Autodesk Fusion 360 part; units mm, degrees
note: some values were not read from the file. Chosen so that the rebuilt part matches the saved one: which bodies a step acts on.
(part 2 of 3)
  line L533 (94.7167, 51.1985) -> (89.24, 51.1985)
  line L534 (89.24, 51.1985) -> (89.24, 52.8883)
  line L535 (89.24, 52.8883) -> (94.5973, 52.8883)
  spline S121 degree 3 poles (94.5973, 52.8883) (96.971, 52.8883) (98.0717, 51.6355) (98.0717, 49.5524) knots 0 0 0 0 1 1 1 1
  spline S122 degree 3 poles (88.5239, 51.0382) (88.5239, 50.5138) (88.1791, 50.1351) (87.7017, 50.1351) knots 0 0 0 0 1 1 1 1
  spline S123 degree 3 poles (87.7017, 50.1351) (87.2243, 50.1351) (86.8796, 50.5138) (86.8796, 51.0382) knots 0 0 0 0 1 1 1 1
  spline S124 degree 3 poles (86.8796, 51.0382) (86.8796, 51.5627) (87.2243, 51.9414) (87.7017, 51.9414) knots 0 0 0 0 1 1 1 1
  spline S125 degree 3 poles (87.7017, 51.9414) (88.1791, 51.9414) (88.5239, 51.5627) (88.5239, 51.0382) knots 0 0 0 0 1 1 1 1
  spline S126 degree 3 poles (88.5239, 48.0956) (88.5239, 47.5712) (88.1791, 47.1925) (87.7017, 47.1925) knots 0 0 0 0 1 1 1 1
  spline S127 degree 3 poles (87.7017, 47.1925) (87.2243, 47.1925) (86.8796, 47.5712) (86.8796, 48.0956) knots 0 0 0 0 1 1 1 1
  spline S128 degree 3 poles (86.8796, 48.0956) (86.8796, 48.6201) (87.2243, 48.9988) (87.7017, 48.9988) knots 0 0 0 0 1 1 1 1
  spline S129 degree 3 poles (87.7017, 48.9988) (88.1791, 48.9988) (88.5239, 48.6201) (88.5239, 48.0956) knots 0 0 0 0 1 1 1 1
  line L536 (97.9126, 35.3898) -> (97.9126, 33.7728)
  line L537 (97.9126, 33.7728) -> (94.12, 33.7728)
  spline S130 degree 3 poles (94.12, 33.7728) (93.1519, 33.7728) (92.1176, 33.9331) (91.1893, 34.0059) knots 0 0 0 0 1 1 1 1
  line L538 (91.1893, 34.0059) -> (91.1893, 33.9622)
  line L539 (91.1893, 33.9622) -> (93.0326, 33.1027)
  line L540 (93.0326, 33.1027) -> (97.9126, 30.5826)
  line L541 (97.9126, 30.5826) -> (97.9126, 28.8054)
  line L542 (97.9126, 28.8054) -> (89.24, 28.8054)
  line L543 (89.24, 28.8054) -> (89.24, 30.4224)
  line L544 (89.24, 30.4224) -> (93.0061, 30.4224)
  spline S131 degree 3 poles (93.0061, 30.4224) (93.9741, 30.4224) (95.0748, 30.2621) (95.9632, 30.1893) knots 0 0 0 0 1 1 1 1
  line L545 (95.9632, 30.1893) -> (95.9632, 30.233)
  line L546 (95.9632, 30.233) -> (94.1067, 31.0925)
  line L547 (94.1067, 31.0925) -> (89.24, 33.6126)
  line L548 (89.24, 33.6126) -> (89.24, 35.3898)
  line L549 (89.24, 35.3898) -> (97.9126, 35.3898)
  line L550 (97.9126, 17.2649) -> (97.9126, 15.5751)
  line L551 (97.9126, 15.5751) -> (94.2924, 15.5751)
  line L552 (94.2924, 15.5751) -> (94.2924, 11.8313)
  line L553 (94.2924, 11.8313) -> (92.9928, 11.8313)
  line L554 (92.9928, 11.8313) -> (92.9928, 15.5751)
  line L555 (92.9928, 15.5751) -> (90.5396, 15.5751)
  line L556 (90.5396, 15.5751) -> (90.5396, 11.1758)
  line L557 (90.5396, 11.1758) -> (89.24, 11.1758)
  line L558 (89.24, 11.1758) -> (89.24, 17.2649)
  line L559 (89.24, 17.2649) -> (97.9126, 17.2649)
  line L560 (116.9551, 192.1915) -> (116.9551, 185.9421)
  line L561 (116.9551, 185.9421) -> (115.6555, 185.9421)
  line L562 (115.6555, 185.9421) -> (115.6555, 190.5017)
  line L563 (115.6555, 190.5017) -> (113.0962, 190.5017)
  line L564 (113.0962, 190.5017) -> (113.0962, 186.7579)
  line L565 (113.0962, 186.7579) -> (111.7966, 186.7579)
  line L566 (111.7966, 186.7579) -> (111.7966, 190.5017)
  line L567 (111.7966, 190.5017) -> (109.5821, 190.5017)
  line L568 (109.5821, 190.5017) -> (109.5821, 186.0878)
  line L569 (109.5821, 186.0878) -> (108.2825, 186.0878)
  line L570 (108.2825, 186.0878) -> (108.2825, 192.1915)
  line L571 (108.2825, 192.1915) -> (116.9551, 192.1915)
  line L572 (116.9551, 174.9989) -> (116.9551, 168.7058)
  line L573 (116.9551, 168.7058) -> (115.6555, 168.7058)
  line L574 (115.6555, 168.7058) -> (115.6555, 171.0075)
  line L575 (115.6555, 171.0075) -> (109.5821, 171.0075)
  line L576 (109.5821, 171.0075) -> (109.5821, 168.7058)
  line L577 (109.5821, 168.7058) -> (108.2825, 168.7058)
  line L578 (108.2825, 168.7058) -> (108.2825, 174.9989)
  line L579 (108.2825, 174.9989) -> (109.5821, 174.9989)
  line L580 (109.5821, 174.9989) -> (109.5821, 172.6973)
  line L581 (109.5821, 172.6973) -> (115.6555, 172.6973)
  line L582 (115.6555, 172.6973) -> (115.6555, 174.9989)
  line L583 (115.6555, 174.9989) -> (116.9551, 174.9989)
  line L584 (116.9551, 157.6752) -> (116.9551, 156.0583)
  line L585 (116.9551, 156.0583) -> (113.1625, 156.0583)
  spline S132 degree 3 poles (113.1625, 156.0583) (112.1944, 156.0583) (111.1601, 156.2185) (110.2318, 156.2913) knots 0 0 0 0 1 1 1 1
  line L586 (110.2318, 156.2913) -> (110.2318, 156.2476)
  line L587 (110.2318, 156.2476) -> (112.0751, 155.3882)
  line L588 (112.0751, 155.3882) -> (116.9551, 152.868)
  line L589 (116.9551, 152.868) -> (116.9551, 151.0908)
  line L590 (116.9551, 151.0908) -> (108.2825, 151.0908)
  line L591 (108.2825, 151.0908) -> (108.2825, 152.7078)
  line L592 (108.2825, 152.7078) -> (112.0486, 152.7078)
  spline S133 degree 3 poles (112.0486, 152.7078) (113.0166, 152.7078) (114.1172, 152.5475) (115.0057, 152.4747) knots 0 0 0 0 1 1 1 1
  line L593 (115.0057, 152.4747) -> (115.0057, 152.5184)
  line L594 (115.0057, 152.5184) -> (113.1492, 153.3779)
  line L595 (113.1492, 153.3779) -> (108.2825, 155.898)
  line L596 (108.2825, 155.898) -> (108.2825, 157.6752)
  line L597 (108.2825, 157.6752) -> (116.9551, 157.6752)
  spline S134 degree 3 poles (117.1142, 136.8845) (117.1142, 134.6703) (115.9472, 133.3593) (114.5416, 133.3593) knots 0 0 0 0 1 1 1 1
  spline S135 degree 3 poles (114.5416, 133.3593) (113.2818, 133.3593) (112.632, 134.2187) (112.1944, 135.4278) knots 0 0 0 0 1 1 1 1
  line L598 (112.1944, 135.4278) -> (111.7038, 136.6806)
  spline S136 degree 3 poles (111.7038, 136.6806) (111.3988, 137.5401) (111.1468, 138.3121) (110.4838, 138.3121) knots 0 0 0 0 1 1 1 1
  spline S137 degree 3 poles (110.4838, 138.3121) (109.834, 138.3121) (109.4627, 137.7003) (109.4627, 136.7971) knots 0 0 0 0 1 1 1 1
  spline S138 degree 3 poles (109.4627, 136.7971) (109.4627, 135.8357) (109.7412, 135.1656) (110.2053, 134.5246) knots 0 0 0 0 1 1 1 1
  line L599 (110.2053, 134.5246) -> (109.224, 133.6506)
  spline S139 degree 3 poles (109.224, 133.6506) (108.5477, 134.4372) (108.1233, 135.5444) (108.1233, 136.7097) knots 0 0 0 0 1 1 1 1
  spline S140 degree 3 poles (108.1233, 136.7097) (108.1233, 138.6472) (109.1842, 140.0165) (110.5633, 140.0165) knots 0 0 0 0 1 1 1 1
  spline S141 degree 3 poles (110.5633, 140.0165) (111.8364, 140.0165) (112.5127, 138.9822) (112.8707, 137.9771) knots 0 0 0 0 1 1 1 1
  line L600 (112.8707, 137.9771) -> (113.3879, 136.6806)
  spline S142 degree 3 poles (113.3879, 136.6806) (113.7459, 135.7338) (113.9581, 135.0782) (114.7272, 135.0782) knots 0 0 0 0 1 1 1 1
  spline S143 degree 3 poles (114.7272, 135.0782) (115.3372, 135.0782) (115.7749, 135.6755) (115.7749, 136.7826) knots 0 0 0 0 1 1 1 1
  spline S144 degree 3 poles (115.7749, 136.7826) (115.7749, 137.7877) (115.377, 138.7346) (114.7935, 139.4484) knots 0 0 0 0 1 1 1 1
  line L601 (114.7935, 139.4484) -> (115.8412, 140.439)
  spline S145 degree 3 poles (115.8412, 140.439) (116.6501, 139.4921) (117.1142, 138.2247) (117.1142, 136.8845) knots 0 0 0 0 1 1 1 1
  line L602 (116.9551, 123.2901) -> (116.9551, 121.4983)
  line L603 (116.9551, 121.4983) -> (114.9129, 120.3038)
  spline S146 degree 3 poles (114.9129, 120.3038) (114.462, 120.0562) (114.0244, 119.8231) (113.494, 119.5609) knots 0 0 0 0 1 1 1 1
  line L604 (113.494, 119.5609) -> (113.494, 119.5026)
  spline S147 degree 3 poles (113.494, 119.5026) (114.0244, 119.2112) (114.462, 118.9636) (114.9129, 118.7014) knots 0 0 0 0 1 1 1 1
  line L605 (114.9129, 118.7014) -> (116.9551, 117.4632)
  line L606 (116.9551, 117.4632) -> (116.9551, 115.5986)
  line L607 (116.9551, 115.5986) -> (112.5525, 118.3955)
  line L608 (112.5525, 118.3955) -> (108.2825, 115.7734)
  line L609 (108.2825, 115.7734) -> (108.2825, 117.5652)
  line L610 (108.2825, 117.5652) -> (110.2053, 118.6431)
  spline S148 degree 3 poles (110.2053, 118.6431) (110.6031, 118.8617) (111.0142, 119.0656) (111.5314, 119.3132) knots 0 0 0 0 1 1 1 1
  line L611 (111.5314, 119.3132) -> (111.5314, 119.3715)
  spline S149 degree 3 poles (111.5314, 119.3715) (111.0142, 119.6628) (110.6031, 119.8813) (110.2053, 120.1144) knots 0 0 0 0 1 1 1 1
  line L612 (110.2053, 120.1144) -> (108.2825, 121.2361)
  line L613 (108.2825, 121.2361) -> (108.2825, 123.1153)
  line L614 (108.2825, 123.1153) -> (112.4862, 120.4932)
  line L615 (112.4862, 120.4932) -> (116.9551, 123.2901)
  spline S150 degree 3 poles (112.3403, 102.8782) (111.4253, 102.5868) (110.444, 102.2955) (109.476, 102.0333) knots 0 0 0 0 1 1 1 1
  line L616 (109.476, 102.0333) -> (109.476, 101.975)
  spline S151 degree 3 poles (109.476, 101.975) (110.444, 101.7128) (111.4253, 101.4069) (112.3403, 101.1301) knots 0 0 0 0 1 1 1 1
  line L617 (112.3403, 101.1301) -> (113.4012, 100.795)
  line L618 (113.4012, 100.795) -> (113.4012, 103.2132)
  line L619 (113.4012, 103.2132) -> (112.3403, 102.8782)
  line L620 (116.9551, 106.0538) -> (116.9551, 104.3349)
  line L621 (116.9551, 104.3349) -> (114.6079, 103.592)
  line L622 (114.6079, 103.592) -> (114.6079, 100.4163)
  line L623 (114.6079, 100.4163) -> (116.9551, 99.6879)
  line L624 (116.9551, 99.6879) -> (116.9551, 97.8961)
  line L625 (116.9551, 97.8961) -> (108.2825, 100.9844)
  line L626 (108.2825, 100.9844) -> (108.2825, 102.9656)
  line L627 (108.2825, 102.9656) -> (116.9551, 106.0538)
  spline S152 degree 3 poles (107.5664, 103.4463) (107.5664, 102.9219) (107.2216, 102.5431) (106.7442, 102.5431) knots 0 0 0 0 1 1 1 1
  spline S153 degree 3 poles (106.7442, 102.5431) (106.2668, 102.5431) (105.9221, 102.9219) (105.9221, 103.4463) knots 0 0 0 0 1 1 1 1
  spline S154 degree 3 poles (105.9221, 103.4463) (105.9221, 103.9707) (106.2668, 104.3495) (106.7442, 104.3495) knots 0 0 0 0 1 1 1 1
  spline S155 degree 3 poles (106.7442, 104.3495) (107.2216, 104.3495) (107.5664, 103.9707) (107.5664, 103.4463) knots 0 0 0 0 1 1 1 1
  spline S156 degree 3 poles (107.5664, 100.5037) (107.5664, 99.9793) (107.2216, 99.6005) (106.7442, 99.6005) knots 0 0 0 0 1 1 1 1
  spline S157 degree 3 poles (106.7442, 99.6005) (106.2668, 99.6005) (105.9221, 99.9793) (105.9221, 100.5037) knots 0 0 0 0 1 1 1 1
  spline S158 degree 3 poles (105.9221, 100.5037) (105.9221, 101.0281) (106.2668, 101.4069) (106.7442, 101.4069) knots 0 0 0 0 1 1 1 1
  spline S159 degree 3 poles (106.7442, 101.4069) (107.2216, 101.4069) (107.5664, 101.0281) (107.5664, 100.5037) knots 0 0 0 0 1 1 1 1
  line L628 (116.9551, 87.929) -> (116.9551, 86.4722)
  line L629 (116.9551, 86.4722) -> (113.4542, 86.4722)
  spline S160 degree 3 poles (113.4542, 86.4722) (112.5392, 86.4722) (110.749, 86.6179) (109.9003, 86.7199) knots 0 0 0 0 1 1 1 1
  line L630 (109.9003, 86.7199) -> (109.9003, 86.6762)
  line L631 (109.9003, 86.6762) -> (111.9159, 86.0498)
  line L632 (111.9159, 86.0498) -> (114.6609, 85.0155)
  line L633 (114.6609, 85.0155) -> (114.6609, 84.0541)
  line L634 (114.6609, 84.0541) -> (111.9159, 83.0052)
  line L635 (111.9159, 83.0052) -> (109.9003, 82.3643)
  line L636 (109.9003, 82.3643) -> (109.9003, 82.3205)
  spline S161 degree 3 poles (109.9003, 82.3205) (110.749, 82.408) (112.5392, 82.5682) (113.4542, 82.5682) knots 0 0 0 0 1 1 1 1
  line L637 (113.4542, 82.5682) -> (116.9551, 82.5682)
  line L638 (116.9551, 82.5682) -> (116.9551, 81.0823)
  line L639 (116.9551, 81.0823) -> (108.2825, 81.0823)
  line L640 (108.2825, 81.0823) -> (108.2825, 82.9469)
  line L641 (108.2825, 82.9469) -> (111.664, 84.0977)
  line L642 (111.664, 84.0977) -> (112.9636, 84.4765)
  line L643 (112.9636, 84.4765) -> (112.9636, 84.5348)
  line L644 (112.9636, 84.5348) -> (111.664, 84.9281)
  line L645 (111.664, 84.9281) -> (108.2825, 86.0643)
  line L646 (108.2825, 86.0643) -> (108.2825, 87.9289)
  line L647 (108.2825, 87.9289) -> (116.9551, 87.929)
  line L648 (116.9551, 70.5179) -> (116.9551, 63.4965)
  line L649 (116.9551, 63.4965) -> (115.6555, 63.4965)
  line L650 (115.6555, 63.4965) -> (115.6555, 68.4493)
  line L651 (115.6555, 68.4493) -> (109.2107, 63.5547)
  line L652 (109.2107, 63.5547) -> (108.2825, 63.5547)
  line L653 (108.2825, 63.5547) -> (108.2825, 70.0809)
  line L654 (108.2825, 70.0809) -> (109.5688, 70.0809)
  line L655 (109.5688, 70.0809) -> (109.5688, 65.6379)
  line L656 (109.5688, 65.6379) -> (116.0268, 70.5179)
  line L657 (116.0268, 70.5179) -> (116.9551, 70.5179)
  line L658 (116.9551, 52.4804) -> (116.9551, 50.6012)
  line L659 (116.9551, 50.6012) -> (113.8785, 49.8729)
  spline S162 degree 3 poles (113.8785, 49.8729) (113.3349, 49.7418) (112.7912, 49.6689) (112.2607, 49.5815) knots 0 0 0 0 1 1 1 1
  line L660 (112.2607, 49.5815) -> (112.2607, 49.5378)
  spline S163 degree 3 poles (112.2607, 49.5378) (112.7912, 49.4795) (113.3349, 49.363) (113.8785, 49.2319) knots 0 0 0 0 1 1 1 1
  line L661 (113.8785, 49.2319) -> (116.9551, 48.489)
  line L662 (116.9551, 48.489) -> (116.9551, 46.5807)
  line L663 (116.9551, 46.5807) -> (108.2825, 45.2988)
  line L664 (108.2825, 45.2988) -> (108.2825, 47.0031)
  line L665 (108.2825, 47.0031) -> (113.3083, 47.4693)
  spline S164 degree 3 poles (113.3083, 47.4693) (114.0244, 47.5275) (114.5681, 47.5421) (115.3903, 47.5858) knots 0 0 0 0 1 1 1 1
  line L666 (115.3903, 47.5858) -> (115.3903, 47.6441)
  spline S165 degree 3 poles (115.3903, 47.6441) (114.5681, 47.7897) (114.0244, 47.9208) (113.3083, 48.1102) knots 0 0 0 0 1 1 1 1
  line L667 (113.3083, 48.1102) -> (110.497, 48.8531)
  line L668 (110.497, 48.8531) -> (110.497, 50.1205)
  line L669 (110.497, 50.1205) -> (113.3083, 50.9071)
  spline S166 degree 3 poles (113.3083, 50.9071) (114.0377, 51.0819) (114.5814, 51.213) (115.3903, 51.3733) knots 0 0 0 0 1 1 1 1
  line L670 (115.3903, 51.3733) -> (115.3903, 51.417)
  spline S167 degree 3 poles (115.3903, 51.417) (114.5814, 51.4461) (114.0377, 51.4898) (113.3083, 51.5481) knots 0 0 0 0 1 1 1 1
  line L671 (113.3083, 51.5481) -> (108.2825, 52.0288)
  line L672 (108.2825, 52.0288) -> (108.2825, 53.8351)
  line L673 (108.2825, 53.8351) -> (116.9551, 52.4804)
  line L674 (116.9551, 34.9674) -> (116.9551, 28.718)
  line L675 (116.9551, 28.718) -> (115.6555, 28.718)
  line L676 (115.6555, 28.718) -> (115.6555, 33.2775)
  line L677 (115.6555, 33.2775) -> (113.0962, 33.2775)
  line L678 (113.0962, 33.2775) -> (113.0962, 29.5337)
  line L679 (113.0962, 29.5337) -> (111.7966, 29.5337)
  line L680 (111.7966, 29.5337) -> (111.7966, 33.2775)
  line L681 (111.7966, 33.2775) -> (109.5821, 33.2775)
  line L682 (109.5821, 33.2775) -> (109.5821, 28.8637)
  line L683 (109.5821, 28.8637) -> (108.2825, 28.8637)
  line L684 (108.2825, 28.8637) -> (108.2825, 34.9674)
  line L685 (108.2825, 34.9674) -> (116.9551, 34.9674)
  line L686 (116.9551, 17.7748) -> (116.9551, 11.4817)
  line L687 (116.9551, 11.4817) -> (115.6555, 11.4817)
  line L688 (115.6555, 11.4817) -> (115.6555, 13.7834)
  line L689 (115.6555, 13.7834) -> (109.5821, 13.7834)
  line L690 (109.5821, 13.7834) -> (109.5821, 11.4817)
  line L691 (109.5821, 11.4817) -> (108.2825, 11.4817)
  line L692 (108.2825, 11.4817) -> (108.2825, 17.7748)
  line L693 (108.2825, 17.7748) -> (109.5821, 17.7748)
  line L694 (109.5821, 17.7748) -> (109.5821, 15.4731)
  line L695 (109.5821, 15.4731) -> (115.6555, 15.4731)
  line L696 (115.6555, 15.4731) -> (115.6555, 17.7748)
  line L697 (115.6555, 17.7748) -> (116.9551, 17.7748)
  line L698 (135.9976, 192.5556) -> (135.9976, 189.9627)
  spline S168 degree 3 poles (135.9976, 189.9627) (135.9976, 187.2386) (134.4991, 185.5634) (131.6215, 185.5634) knots 0 0 0 0 1 1 1 1
  spline S169 degree 3 poles (131.6215, 185.5634) (128.7572, 185.5634) (127.325, 187.2386) (127.325, 190.0501) knots 0 0 0 0 1 1 1 1
  line L699 (127.325, 190.0501) -> (127.325, 192.5556)
  line L700 (127.325, 192.5556) -> (135.9976, 192.5556)
  line L701 (134.751, 190.8658) -> (128.5715, 190.8658)
  line L702 (128.5715, 190.8658) -> (128.5715, 190.152)
  spline S170 degree 3 poles (128.5715, 190.152) (128.5715, 188.3311) (129.4997, 187.2969) (131.6215, 187.2969) knots 0 0 0 0 1 1 1 1
  spline S171 degree 3 poles (131.6215, 187.2969) (133.7565, 187.2969) (134.751, 188.3311) (134.751, 190.152) knots 0 0 0 0 1 1 1 1
  line L703 (134.751, 190.152) -> (134.751, 190.8658)
  line L704 (135.9976, 174.9989) -> (135.9976, 173.3091)
  line L705 (135.9976, 173.3091) -> (132.6028, 173.3091)
  line L706 (132.6028, 173.3091) -> (132.6028, 171.8815)
  line L707 (132.6028, 171.8815) -> (135.9976, 169.8421)
  line L708 (135.9976, 169.8421) -> (135.9976, 167.9338)
  line L709 (135.9976, 167.9338) -> (132.3773, 170.2063)
  spline S172 degree 3 poles (132.3773, 170.2063) (132.0193, 169.07) (131.2104, 168.3125) (129.8976, 168.3125) knots 0 0 0 0 1 1 1 1
  spline S173 degree 3 poles (129.8976, 168.3125) (127.9615, 168.3125) (127.325, 169.8421) (127.325, 171.8232) knots 0 0 0 0 1 1 1 1
  line L710 (127.325, 171.8232) -> (127.325, 174.9989)
  line L711 (127.325, 174.9989) -> (135.9976, 174.9989)
  line L712 (131.3828, 173.3091) -> (128.5582, 173.3091)
  line L713 (128.5582, 173.3091) -> (128.5582, 171.998)
  spline S174 degree 3 poles (128.5582, 171.998) (128.5582, 170.687) (128.903, 169.9732) (129.8976, 169.9732) knots 0 0 0 0 1 1 1 1
  spline S175 degree 3 poles (129.8976, 169.9732) (130.8789, 169.9732) (131.3828, 170.687) (131.3828, 171.998) knots 0 0 0 0 1 1 1 1
  line L714 (131.3828, 171.998) -> (131.3828, 173.3091)
  line L715 (135.9976, 157.2528) -> (135.9976, 151.0034)
  line L716 (135.9976, 151.0034) -> (134.698, 151.0034)
  line L717 (134.698, 151.0034) -> (134.698, 155.563)
  line L718 (134.698, 155.563) -> (132.1386, 155.563)
  line L719 (132.1386, 155.563) -> (132.1386, 151.8192)
  line L720 (132.1386, 151.8192) -> (130.8391, 151.8192)
  line L721 (130.8391, 151.8192) -> (130.8391, 155.563)
  line L722 (130.8391, 155.563) -> (128.6245, 155.563)
  line L723 (128.6245, 155.563) -> (128.6245, 151.1491)
  line L724 (128.6245, 151.1491) -> (127.325, 151.1491)
  line L725 (127.325, 151.1491) -> (127.325, 157.2528)
  line L726 (127.325, 157.2528) -> (135.9976, 157.2528)
  line L727 (135.9976, 140.0602) -> (135.9976, 133.7672)
  line L728 (135.9976, 133.7672) -> (134.698, 133.7672)
  line L729 (134.698, 133.7672) -> (134.698, 136.0688)
  line L730 (134.698, 136.0688) -> (128.6245, 136.0688)
  line L731 (128.6245, 136.0688) -> (128.6245, 133.7672)
  line L732 (128.6245, 133.7672) -> (127.325, 133.7672)
  line L733 (127.325, 133.7672) -> (127.325, 140.0602)
  line L734 (127.325, 140.0602) -> (128.6245, 140.0602)
  line L735 (128.6245, 140.0602) -> (128.6245, 137.7586)
  line L736 (128.6245, 137.7586) -> (134.698, 137.7586)
  line L737 (134.698, 137.7586) -> (134.698, 140.0602)
  line L738 (134.698, 140.0602) -> (135.9976, 140.0602)
  spline S176 degree 3 poles (131.3828, 120.3475) (130.4678, 120.0562) (129.4865, 119.7648) (128.5185, 119.5026) knots 0 0 0 0 1 1 1 1
  line L739 (128.5185, 119.5026) -> (128.5185, 119.4443)
  spline S177 degree 3 poles (128.5185, 119.4443) (129.4865, 119.1821) (130.4678, 118.8762) (131.3828, 118.5994) knots 0 0 0 0 1 1 1 1
  line L740 (131.3828, 118.5994) -> (132.4437, 118.2644)
  line L741 (132.4437, 118.2644) -> (132.4437, 120.6825)
  line L742 (132.4437, 120.6825) -> (131.3828, 120.3475)
  line L743 (135.9976, 123.5232) -> (135.9976, 121.8042)
  line L744 (135.9976, 121.8042) -> (133.6504, 121.0613)
  line L745 (133.6504, 121.0613) -> (133.6504, 117.8856)
  line L746 (133.6504, 117.8856) -> (135.9976, 117.1573)
  line L747 (135.9976, 117.1573) -> (135.9976, 115.3655)
  line L748 (135.9976, 115.3655) -> (127.325, 118.4538)
  line L749 (127.325, 118.4538) -> (127.325, 120.4349)
  line L750 (127.325, 120.4349) -> (135.9976, 123.5232)
  spline S178 degree 3 poles (136.1567, 101.9604) (136.1567, 99.8627) (135.0561, 98.6537) (132.6823, 98.6537) knots 0 0 0 0 1 1 1 1
  line L751 (132.6823, 98.6537) -> (127.325, 98.6537)
  line L752 (127.325, 98.6537) -> (127.325, 100.2706)
  line L753 (127.325, 100.2706) -> (132.8017, 100.2706)
  spline S179 degree 3 poles (132.8017, 100.2706) (134.2206, 100.2706) (134.8173, 100.9261) (134.8173, 101.9604) knots 0 0 0 0 1 1 1 1
  spline S180 degree 3 poles (134.8173, 101.9604) (134.8173, 102.9801) (134.2206, 103.6065) (132.8017, 103.6065) knots 0 0 0 0 1 1 1 1
  line L754 (132.8017, 103.6065) -> (127.325, 103.6065)
  line L755 (127.325, 103.6065) -> (127.325, 105.2963)
  line L756 (127.325, 105.2963) -> (132.6823, 105.2963)
  spline S181 degree 3 poles (132.6823, 105.2963) (135.056, 105.2963) (136.1567, 104.0435) (136.1567, 101.9604) knots 0 0 0 0 1 1 1 1
  spline S182 degree 3 poles (136.1567, 84.8844) (136.1567, 82.3788) (134.7908, 81.5194) (133.1332, 81.5194) knots 0 0 0 0 1 1 1 1
  line L757 (133.1332, 81.5194) -> (127.325, 81.5194)
  line L758 (127.325, 81.5194) -> (127.325, 87.0695)
  line L759 (127.325, 87.0695) -> (128.6113, 87.0695)
  line L760 (128.6113, 87.0695) -> (128.6113, 83.2092)
  line L761 (128.6113, 83.2092) -> (133.0006, 83.2092)
  spline S183 degree 3 poles (133.0006, 83.2092) (134.3135, 83.2092) (134.8174, 83.7627) (134.8174, 84.9281) knots 0 0 0 0 1 1 1 1
  spline S184 degree 3 poles (134.8174, 84.9281) (134.8174, 85.6128) (134.4726, 86.312) (133.7698, 86.8656) knots 0 0 0 0 1 1 1 1
  line L762 (133.7698, 86.8656) -> (134.7245, 87.8561)
  spline S185 degree 3 poles (134.7245, 87.8561) (135.7456, 87.1132) (136.1567, 85.9333) (136.1567, 84.8844) knots 0 0 0 0 1 1 1 1
  line L763 (135.9976, 68.0269) -> (135.9976, 66.0312)
  line L764 (135.9976, 66.0312) -> (127.325, 63.074)
  line L765 (127.325, 63.074) -> (127.325, 64.8075)
  line L766 (127.325, 64.8075) -> (131.6878, 66.1331)
  spline S186 degree 3 poles (131.6878, 66.1331) (132.6691, 66.4245) (133.5178, 66.643) (134.5123, 66.9635) knots 0 0 0 0 1 1 1 1
  line L767 (134.5123, 66.9635) -> (134.5123, 67.0218)
  spline S187 degree 3 poles (134.5123, 67.0218) (133.5178, 67.3422) (132.6691, 67.5608) (131.6878, 67.8667) knots 0 0 0 0 1 1 1 1
  line L768 (131.6878, 67.8667) -> (127.325, 69.2068)
  line L769 (127.325, 69.2068) -> (127.325, 70.9986)
  line L770 (127.325, 70.9986) -> (135.9976, 68.0269)
  line L771 (135.9976, 52.7135) -> (135.9976, 46.4204)
  line L772 (135.9976, 46.4204) -> (134.698, 46.4204)
  line L773 (134.698, 46.4204) -> (134.698, 48.7221)
  line L774 (134.698, 48.7221) -> (128.6245, 48.7221)
  line L775 (128.6245, 48.7221) -> (128.6245, 46.4204)
  line L776 (128.6245, 46.4204) -> (127.325, 46.4204)
  line L777 (127.325, 46.4204) -> (127.325, 52.7135)
  line L778 (127.325, 52.7135) -> (128.6245, 52.7135)
  line L779 (128.6245, 52.7135) -> (128.6245, 50.4119)
  line L780 (128.6245, 50.4119) -> (134.698, 50.4119)
  line L781 (134.698, 50.4119) -> (134.698, 52.7135)
  line L782 (134.698, 52.7135) -> (135.9976, 52.7135)
  line L783 (135.9976, 34.9674) -> (135.9976, 28.718)
  line L784 (135.9976, 28.718) -> (134.698, 28.718)
  line L785 (134.698, 28.718) -> (134.698, 33.2775)
  line L786 (134.698, 33.2775) -> (132.1386, 33.2775)
  line L787 (132.1386, 33.2775) -> (132.1386, 29.5337)
  line L788 (132.1386, 29.5337) -> (130.8391, 29.5337)
  line L789 (130.8391, 29.5337) -> (130.8391, 33.2775)
  line L790 (130.8391, 33.2775) -> (128.6245, 33.2775)
  line L791 (128.6245, 33.2775) -> (128.6245, 28.8637)
  line L792 (128.6245, 28.8637) -> (127.325, 28.8637)
  line L793 (127.325, 28.8637) -> (127.325, 34.9674)
  line L794 (127.325, 34.9674) -> (135.9976, 34.9674)
  line L795 (135.9976, 17.7748) -> (135.9976, 16.085)
  line L796 (135.9976, 16.085) -> (132.6028, 16.085)
  line L797 (132.6028, 16.085) -> (132.6028, 14.6574)
  line L798 (132.6028, 14.6574) -> (135.9976, 12.618)
  line L799 (135.9976, 12.618) -> (135.9976, 10.7096)
  line L800 (135.9976, 10.7096) -> (132.3773, 12.9822)
  spline S188 degree 3 poles (132.3773, 12.9822) (132.0193, 11.8459) (131.2104, 11.0884) (129.8976, 11.0884) knots 0 0 0 0 1 1 1 1
  spline S189 degree 3 poles (129.8976, 11.0884) (127.9615, 11.0884) (127.325, 12.618) (127.325, 14.5991) knots 0 0 0 0 1 1 1 1
  line L801 (127.325, 14.5991) -> (127.325, 17.7748)
  line L802 (127.325, 17.7748) -> (135.9976, 17.7748)
  line L803 (131.3828, 16.085) -> (128.5582, 16.085)
  line L804 (128.5582, 16.085) -> (128.5582, 14.7739)
  spline S190 degree 3 poles (128.5582, 14.7739) (128.5582, 13.4629) (128.903, 12.7491) (129.8976, 12.7491) knots 0 0 0 0 1 1 1 1
  spline S191 degree 3 poles (129.8976, 12.7491) (130.8789, 12.7491) (131.3828, 13.4628) (131.3828, 14.7739) knots 0 0 0 0 1 1 1 1
  line L805 (131.3828, 14.7739) -> (131.3828, 16.085)
  spline S192 degree 3 poles (155.1992, 189.2926) (155.1992, 187.0784) (154.0322, 185.7673) (152.6266, 185.7673) knots 0 0 0 0 1 1 1 1
  spline S193 degree 3 poles (152.6266, 185.7673) (151.3668, 185.7673) (150.717, 186.6268) (150.2794, 187.8358) knots 0 0 0 0 1 1 1 1
  line L806 (150.2794, 187.8358) -> (149.7888, 189.0886)
  spline S194 degree 3 poles (149.7888, 189.0886) (149.4838, 189.9481) (149.2318, 190.7202) (148.5688, 190.7202) knots 0 0 0 0 1 1 1 1
  spline S195 degree 3 poles (148.5688, 190.7202) (147.919, 190.7202) (147.5477, 190.1083) (147.5477, 189.2052) knots 0 0 0 0 1 1 1 1
  spline S196 degree 3 poles (147.5477, 189.2052) (147.5477, 188.2437) (147.8262, 187.5736) (148.2903, 186.9327) knots 0 0 0 0 1 1 1 1
  line L807 (148.2903, 186.9327) -> (147.309, 186.0586)
  spline S197 degree 3 poles (147.309, 186.0586) (146.6327, 186.8453) (146.2083, 187.9524) (146.2083, 189.1178) knots 0 0 0 0 1 1 1 1
  spline S198 degree 3 poles (146.2083, 189.1178) (146.2083, 191.0552) (147.2692, 192.4245) (148.6483, 192.4245) knots 0 0 0 0 1 1 1 1
  spline S199 degree 3 poles (148.6483, 192.4245) (149.9214, 192.4245) (150.5977, 191.3903) (150.9557, 190.3851) knots 0 0 0 0 1 1 1 1
  line L808 (150.9557, 190.3851) -> (151.4729, 189.0886)
  spline S200 degree 3 poles (151.4729, 189.0886) (151.8309, 188.1418) (152.0431, 187.4862) (152.8122, 187.4862) knots 0 0 0 0 1 1 1 1
  spline S201 degree 3 poles (152.8122, 187.4862) (153.4222, 187.4862) (153.8598, 188.0835) (153.8598, 189.1906) knots 0 0 0 0 1 1 1 1
  spline S202 degree 3 poles (153.8598, 189.1906) (153.8598, 190.1957) (153.462, 191.1426) (152.8785, 191.8564) knots 0 0 0 0 1 1 1 1
  line L809 (152.8785, 191.8564) -> (153.9262, 192.847)
  spline S203 degree 3 poles (153.9262, 192.847) (154.735, 191.9001) (155.1992, 190.6327) (155.1992, 189.2926) knots 0 0 0 0 1 1 1 1
  line L810 (155.04, 174.7221) -> (155.04, 168.4728)
  line L811 (155.04, 168.4728) -> (153.7405, 168.4728)
  line L812 (153.7405, 168.4728) -> (153.7405, 173.0323)
  line L813 (153.7405, 173.0323) -> (151.1811, 173.0323)
  line L814 (151.1811, 173.0323) -> (151.1811, 169.2885)
  line L815 (151.1811, 169.2885) -> (149.8816, 169.2885)
  line L816 (149.8816, 169.2885) -> (149.8816, 173.0323)
  line L817 (149.8816, 173.0323) -> (147.667, 173.0323)
  line L818 (147.667, 173.0323) -> (147.667, 168.6184)
  line L819 (147.667, 168.6184) -> (146.3674, 168.6184)
  line L820 (146.3674, 168.6184) -> (146.3674, 174.7221)
  line L821 (146.3674, 174.7221) -> (155.04, 174.7221)
  spline S204 degree 3 poles (155.1992, 153.5964) (155.1992, 152.329) (154.7483, 151.3239) (153.9394, 150.5664) knots 0 0 0 0 1 1 1 1
  line L822 (153.9394, 150.5664) -> (152.9979, 151.4987)
  spline S205 degree 3 poles (152.9979, 151.4987) (153.5416, 152.0377) (153.8598, 152.6641) (153.8598, 153.4362) knots 0 0 0 0 1 1 1 1
  spline S206 degree 3 poles (153.8598, 153.4362) (153.8598, 155.0677) (152.6664, 156.1457) (150.6905, 156.1457) knots 0 0 0 0 1 1 1 1
  spline S207 degree 3 poles (150.6905, 156.1457) (148.7412, 156.1457) (147.5477, 155.0677) (147.5477, 153.4799) knots 0 0 0 0 1 1 1 1
  spline S208 degree 3 poles (147.5477, 153.4799) (147.5477, 152.7369) (147.8262, 152.1688) (148.2505, 151.6881) knots 0 0 0 0 1 1 1 1
  line L823 (148.2505, 151.6881) -> (147.2957, 150.7558)
  spline S209 degree 3 poles (147.2957, 150.7558) (146.7255, 151.353) (146.2083, 152.2999) (146.2083, 153.4799) knots 0 0 0 0 1 1 1 1
  spline S210 degree 3 poles (146.2083, 153.4799) (146.2083, 156) (147.8924, 157.8792) (150.7302, 157.8792) knots 0 0 0 0 1 1 1 1
  spline S211 degree 3 poles (150.7302, 157.8792) (153.6078, 157.8792) (155.1991, 155.9563) (155.1992, 153.5964) knots 0 0 0 0 1 1 1 1
  line L824 (155.04, 140.235) -> (155.04, 138.5452)
  line L825 (155.04, 138.5452) -> (151.1944, 138.5452)
  line L826 (151.1944, 138.5452) -> (151.1944, 135.2822)
  line L827 (151.1944, 135.2822) -> (155.04, 135.2822)
  line L828 (155.04, 135.2822) -> (155.04, 133.5924)
  line L829 (155.04, 133.5924) -> (146.3675, 133.5924)
  line L830 (146.3675, 133.5924) -> (146.3675, 135.2822)
  line L831 (146.3675, 135.2822) -> (149.8551, 135.2822)
  line L832 (149.8551, 135.2822) -> (149.8551, 138.5452)
  line L833 (149.8551, 138.5452) -> (146.3675, 138.5452)
  line L834 (146.3675, 138.5452) -> (146.3675, 140.235)
  line L835 (146.3675, 140.235) -> (155.04, 140.235)
  spline S212 degree 3 poles (155.1992, 119.4152) (155.1992, 117.201) (154.0322, 115.8899) (152.6266, 115.8899) knots 0 0 0 0 1 1 1 1
  spline S213 degree 3 poles (152.6266, 115.8899) (151.3668, 115.8899) (150.717, 116.7494) (150.2794, 117.9585) knots 0 0 0 0 1 1 1 1
  line L836 (150.2794, 117.9585) -> (149.7888, 119.2113)
  spline S214 degree 3 poles (149.7888, 119.2113) (149.4838, 120.0707) (149.2318, 120.8428) (148.5688, 120.8428) knots 0 0 0 0 1 1 1 1
  spline S215 degree 3 poles (148.5688, 120.8428) (147.919, 120.8428) (147.5477, 120.231) (147.5477, 119.3278) knots 0 0 0 0 1 1 1 1
  spline S216 degree 3 poles (147.5477, 119.3278) (147.5477, 118.3664) (147.8262, 117.6963) (148.2903, 117.0553) knots 0 0 0 0 1 1 1 1
  line L837 (148.2903, 117.0553) -> (147.309, 116.1813)
  spline S217 degree 3 poles (147.309, 116.1813) (146.6327, 116.9679) (146.2083, 118.075) (146.2083, 119.2404) knots 0 0 0 0 1 1 1 1
  spline S218 degree 3 poles (146.2083, 119.2404) (146.2083, 121.1779) (147.2692, 122.5472) (148.6483, 122.5472) knots 0 0 0 0 1 1 1 1
  spline S219 degree 3 poles (148.6483, 122.5472) (149.9214, 122.5472) (150.5977, 121.5129) (150.9557, 120.5078) knots 0 0 0 0 1 1 1 1
  line L838 (150.9557, 120.5078) -> (151.4729, 119.2113)
  spline S220 degree 3 poles (151.4729, 119.2113) (151.8309, 118.2644) (152.0431, 117.6089) (152.8122, 117.6089) knots 0 0 0 0 1 1 1 1
  spline S221 degree 3 poles (152.8122, 117.6089) (153.4222, 117.6089) (153.8598, 118.2061) (153.8598, 119.3133) knots 0 0 0 0 1 1 1 1
  spline S222 degree 3 poles (153.8598, 119.3133) (153.8598, 120.3184) (153.462, 121.2653) (152.8785, 121.9791) knots 0 0 0 0 1 1 1 1
  line L839 (152.8785, 121.9791) -> (153.9262, 122.9696)
  spline S223 degree 3 poles (153.9262, 122.9696) (154.735, 122.0228) (155.1992, 120.7554) (155.1992, 119.4152) knots 0 0 0 0 1 1 1 1
  line L840 (155.04, 105.2672) -> (155.04, 103.6502)
  line L841 (155.04, 103.6502) -> (151.2474, 103.6502)
  spline S224 degree 3 poles (151.2474, 103.6502) (150.2794, 103.6502) (149.2451, 103.8105) (148.3168, 103.8833) knots 0 0 0 0 1 1 1 1
  line L842 (148.3168, 103.8833) -> (148.3168, 103.8396)
  line L843 (148.3168, 103.8396) -> (150.1601, 102.9801)
  line L844 (150.1601, 102.9801) -> (155.04, 100.46)
  line L845 (155.04, 100.46) -> (155.04, 98.6828)
  line L846 (155.04, 98.6828) -> (146.3675, 98.6828)
  line L847 (146.3675, 98.6828) -> (146.3675, 100.2997)
  line L848 (146.3675, 100.2997) -> (150.1335, 100.2997)
  spline S225 degree 3 poles (150.1335, 100.2997) (151.1016, 100.2997) (152.2022, 100.1395) (153.0907, 100.0667) knots 0 0 0 0 1 1 1 1
  line L849 (153.0907, 100.0667) -> (153.0907, 100.1104)
  line L850 (153.0907, 100.1104) -> (151.2342, 100.9699)
  line L851 (151.2342, 100.9699) -> (146.3675, 103.49)
  line L852 (146.3675, 103.49) -> (146.3675, 105.2672)
  line L853 (146.3675, 105.2672) -> (155.04, 105.2672)
  line L854 (155.04, 87.1278) -> (155.04, 80.9804)
  line L855 (155.04, 80.9804) -> (153.7405, 80.9804)
  line L856 (153.7405, 80.9804) -> (153.7405, 85.4525)
  line L857 (153.7405, 85.4525) -> (146.3675, 85.4525)
  line L858 (146.3675, 85.4525) -> (146.3675, 87.1278)
  line L859 (146.3675, 87.1278) -> (155.04, 87.1278)
  spline S226 degree 3 poles (150.4253, 67.9395) (149.5103, 67.6481) (148.529, 67.3568) (147.561, 67.0946) knots 0 0 0 0 1 1 1 1
  line L860 (147.561, 67.0946) -> (147.561, 67.0363)
  spline S227 degree 3 poles (147.561, 67.0363) (148.529, 66.7741) (149.5103, 66.4682) (150.4253, 66.1914) knots 0 0 0 0 1 1 1 1
  line L861 (150.4253, 66.1914) -> (151.4861, 65.8564)
  line L862 (151.4861, 65.8564) -> (151.4861, 68.2745)
  line L863 (151.4861, 68.2745) -> (150.4253, 67.9395)
  line L864 (155.04, 71.1152) -> (155.04, 69.3962)
  line L865 (155.04, 69.3962) -> (152.6929, 68.6533)
  line L866 (152.6929, 68.6533) -> (152.6929, 65.4776)
  line L867 (152.6929, 65.4776) -> (155.04, 64.7492)
  line L868 (155.04, 64.7492) -> (155.04, 62.9575)
  line L869 (155.04, 62.9575) -> (146.3675, 66.0457)
  line L870 (146.3675, 66.0457) -> (146.3675, 68.0269)
  line L871 (146.3675, 68.0269) -> (155.04, 71.1152)
  spline S228 degree 3 poles (155.1992, 48.7803) (155.1992, 47.513) (154.7483, 46.5078) (153.9394, 45.7503) knots 0 0 0 0 1 1 1 1
  line L872 (153.9394, 45.7503) -> (152.9979, 46.6826)
  spline S229 degree 3 poles (152.9979, 46.6826) (153.5416, 47.2216) (153.8598, 47.848) (153.8598, 48.6201) knots 0 0 0 0 1 1 1 1
  spline S230 degree 3 poles (153.8598, 48.6201) (153.8598, 50.2516) (152.6664, 51.3296) (150.6905, 51.3296) knots 0 0 0 0 1 1 1 1
  spline S231 degree 3 poles (150.6905, 51.3296) (148.7412, 51.3296) (147.5477, 50.2516) (147.5477, 48.6637) knots 0 0 0 0 1 1 1 1
  spline S232 degree 3 poles (147.5477, 48.6637) (147.5477, 47.9208) (147.8262, 47.3527) (148.2505, 46.872) knots 0 0 0 0 1 1 1 1
  line L873 (148.2505, 46.872) -> (147.2957, 45.9397)
  spline S233 degree 3 poles (147.2957, 45.9397) (146.7255, 46.5369) (146.2083, 47.4838) (146.2083, 48.6637) knots 0 0 0 0 1 1 1 1
  spline S234 degree 3 poles (146.2083, 48.6637) (146.2083, 51.1839) (147.8924, 53.0631) (150.7302, 53.0631) knots 0 0 0 0 1 1 1 1
  spline S235 degree 3 poles (150.7302, 53.0631) (153.6078, 53.0631) (155.1991, 51.1402) (155.1992, 48.7803) knots 0 0 0 0 1 1 1 1
  line L874 (155.04, 35.419) -> (155.04, 33.7292)
  line L875 (155.04, 33.7292) -> (151.1944, 33.7292)
  line L876 (151.1944, 33.7292) -> (151.1944, 30.4661)
  line L877 (151.1944, 30.4661) -> (155.04, 30.4661)
  line L878 (155.04, 30.4661) -> (155.04, 28.7763)
  line L879 (155.04, 28.7763) -> (146.3675, 28.7763)
  line L880 (146.3675, 28.7763) -> (146.3675, 30.4661)
  line L881 (146.3675, 30.4661) -> (149.8551, 30.4661)
  line L882 (149.8551, 30.4661) -> (149.8551, 33.7292)
  line L883 (149.8551, 33.7292) -> (146.3675, 33.7292)
  line L884 (146.3675, 33.7292) -> (146.3675, 35.419)
  line L885 (146.3675, 35.419) -> (155.04, 35.419)
  line L886 (155.04, 15.4732) -> (155.04, 13.7834)
  line L887 (155.04, 13.7834) -> (147.667, 13.7834)
  line L888 (147.667, 13.7834) -> (147.667, 10.7825)
  line L889 (147.667, 10.7825) -> (146.3675, 10.7825)
  line L890 (146.3675, 10.7825) -> (146.3675, 18.4741)
  line L891 (146.3675, 18.4741) -> (147.667, 18.4741)
  line L892 (147.667, 18.4741) -> (147.667, 15.4732)
  line L893 (147.667, 15.4732) -> (155.04, 15.4732)
  spline S236 degree 3 poles (174.2417, 189.2926) (174.2417, 187.0784) (173.0747, 185.7673) (171.6691, 185.7673) knots 0 0 0 0 1 1 1 1
  spline S237 degree 3 poles (171.6691, 185.7673) (170.4093, 185.7673) (169.7595, 186.6268) (169.3219, 187.8358) knots 0 0 0 0 1 1 1 1
  line L894 (169.3219, 187.8358) -> (168.8313, 189.0886)
  spline S238 degree 3 poles (168.8313, 189.0886) (168.5263, 189.9481) (168.2743, 190.7202) (167.6113, 190.7202) knots 0 0 0 0 1 1 1 1
  spline S239 degree 3 poles (167.6113, 190.7202) (166.9615, 190.7202) (166.5902, 190.1083) (166.5902, 189.2052) knots 0 0 0 0 1 1 1 1
  spline S240 degree 3 poles (166.5902, 189.2052) (166.5902, 188.2437) (166.8687, 187.5736) (167.3328, 186.9327) knots 0 0 0 0 1 1 1 1
  line L895 (167.3328, 186.9327) -> (166.3515, 186.0586)
  spline S241 degree 3 poles (166.3515, 186.0586) (165.6752, 186.8453) (165.2509, 187.9524) (165.2509, 189.1178) knots 0 0 0 0 1 1 1 1
  spline S242 degree 3 poles (165.2509, 189.1178) (165.2509, 191.0552) (166.3117, 192.4245) (167.6909, 192.4245) knots 0 0 0 0 1 1 1 1
  spline S243 degree 3 poles (167.6909, 192.4245) (168.9639, 192.4245) (169.6402, 191.3903) (169.9982, 190.3851) knots 0 0 0 0 1 1 1 1
  line L896 (169.9982, 190.3851) -> (170.5154, 189.0886)
  spline S244 degree 3 poles (170.5154, 189.0886) (170.8735, 188.1418) (171.0856, 187.4862) (171.8548, 187.4862) knots 0 0 0 0 1 1 1 1
  spline S245 degree 3 poles (171.8548, 187.4862) (172.4648, 187.4862) (172.9024, 188.0835) (172.9024, 189.1906) knots 0 0 0 0 1 1 1 1
  spline S246 degree 3 poles (172.9024, 189.1906) (172.9024, 190.1957) (172.5045, 191.1426) (171.9211, 191.8564) knots 0 0 0 0 1 1 1 1
  line L897 (171.9211, 191.8564) -> (172.9687, 192.847)
  spline S247 degree 3 poles (172.9687, 192.847) (173.7776, 191.9001) (174.2417, 190.6327) (174.2417, 189.2926) knots 0 0 0 0 1 1 1 1
  line L898 (174.0825, 174.9989) -> (174.0825, 168.7058)
  line L899 (174.0825, 168.7058) -> (172.783, 168.7058)
  line L900 (172.783, 168.7058) -> (172.783, 171.0075)
  line L901 (172.783, 171.0075) -> (166.7095, 171.0075)
  line L902 (166.7095, 171.0075) -> (166.7095, 168.7058)
  line L903 (166.7095, 168.7058) -> (165.41, 168.7058)
  line L904 (165.41, 168.7058) -> (165.41, 174.9989)
  line L905 (165.41, 174.9989) -> (166.7095, 174.9989)
  line L906 (166.7095, 174.9989) -> (166.7095, 172.6973)
  line L907 (166.7095, 172.6973) -> (172.783, 172.6973)
  line L908 (172.783, 172.6973) -> (172.783, 174.9989)
  line L909 (172.783, 174.9989) -> (174.0825, 174.9989)
  line L910 (174.0825, 157.2528) -> (174.0825, 151.0034)
  line L911 (174.0825, 151.0034) -> (172.783, 151.0034)
  line L912 (172.783, 151.0034) -> (172.783, 155.563)
  line L913 (172.783, 155.563) -> (170.2236, 155.563)
  line L914 (170.2236, 155.563) -> (170.2236, 151.8192)
  line L915 (170.2236, 151.8192) -> (168.9241, 151.8192)
  line L916 (168.9241, 151.8192) -> (168.9241, 155.563)
  line L917 (168.9241, 155.563) -> (166.7095, 155.563)
  line L918 (166.7095, 155.563) -> (166.7095, 151.1491)
  line L919 (166.7095, 151.1491) -> (165.41, 151.1491)
  line L920 (165.41, 151.1491) -> (165.41, 157.2528)
  line L921 (165.41, 157.2528) -> (174.0825, 157.2528)
  line L922 (174.0825, 140.0311) -> (174.0825, 136.8263)
  spline S248 degree 3 poles (174.0825, 136.8263) (174.0825, 134.7286) (173.2736, 133.199) (171.5365, 133.199) knots 0 0 0 0 1 1 1 1
  spline S249 degree 3 poles (171.5365, 133.199) (170.3563, 133.199) (169.6932, 133.9711) (169.481, 135.3404) knots 0 0 0 0 1 1 1 1
  line L923 (169.481, 135.3404) -> (169.428, 135.3404)
  spline S250 degree 3 poles (169.428, 135.3404) (169.1628, 134.2187) (168.3671, 133.6943) (167.545, 133.6943) knots 0 0 0 0 1 1 1 1
  spline S251 degree 3 poles (167.545, 133.6943) (165.9537, 133.6943) (165.41, 135.1074) (165.41, 137.0739) knots 0 0 0 0 1 1 1 1
  line L924 (165.41, 137.0739) -> (165.41, 140.0311)
  line L925 (165.41, 140.0311) -> (174.0825, 140.0311)
  line L926 (168.9771, 138.3413) -> (166.6432, 138.3413)
  line L927 (166.6432, 138.3413) -> (166.6432, 137.1905)
  spline S252 degree 3 poles (166.6432, 137.1905) (166.6432, 135.9522) (166.935, 135.355) (167.7306, 135.355) knots 0 0 0 0 1 1 1 1
  spline S253 degree 3 poles (167.7306, 135.355) (168.5395, 135.355) (168.9771, 135.894) (168.9771, 137.2196) knots 0 0 0 0 1 1 1 1
  line L928 (168.9771, 137.2196) -> (168.9771, 138.3413)
  line L929 (172.8493, 138.3413) -> (170.1441, 138.3413)
  line L930 (170.1441, 138.3413) -> (170.1441, 137.0011)
  spline S254 degree 3 poles (170.1441, 137.0011) (170.1441, 135.5735) (170.5154, 134.8597) (171.4304, 134.8597) knots 0 0 0 0 1 1 1 1
  spline S255 degree 3 poles (171.4304, 134.8597) (172.4117, 134.8597) (172.8493, 135.6026) (172.8493, 137.0011) knots 0 0 0 0 1 1 1 1
  line L931 (172.8493, 137.0011) -> (172.8493, 138.3413)
  line L932 (174.0825, 122.3141) -> (174.0825, 116.0647)
  line L933 (174.0825, 116.0647) -> (172.783, 116.0647)
  line L934 (172.783, 116.0647) -> (172.783, 120.6243)
  line L935 (172.783, 120.6243) -> (170.2236, 120.6243)
  line L936 (170.2236, 120.6243) -> (170.2236, 116.8805)
  line L937 (170.2236, 116.8805) -> (168.9241, 116.8805)
  line L938 (168.9241, 116.8805) -> (168.9241, 120.6243)
  line L939 (168.9241, 120.6243) -> (166.7095, 120.6243)
  line L940 (166.7095, 120.6243) -> (166.7095, 116.2104)
  line L941 (166.7095, 116.2104) -> (165.41, 116.2104)
  line L942 (165.41, 116.2104) -> (165.41, 122.3141)
  line L943 (165.41, 122.3141) -> (174.0825, 122.3141)
  line L944 (174.0825, 105.2672) -> (174.0825, 103.6502)
  line L945 (174.0825, 103.6502) -> (170.2899, 103.6502)
  spline S256 degree 3 poles (170.2899, 103.6502) (169.3219, 103.6502) (168.2876, 103.8105) (167.3593, 103.8833) knots 0 0 0 0 1 1 1 1
  line L946 (167.3593, 103.8833) -> (167.3593, 103.8396)
  line L947 (167.3593, 103.8396) -> (169.2026, 102.9801)
  line L948 (169.2026, 102.9801) -> (174.0825, 100.46)
  line L949 (174.0825, 100.46) -> (174.0825, 98.6828)
  line L950 (174.0825, 98.6828) -> (165.41, 98.6828)
  line L951 (165.41, 98.6828) -> (165.41, 100.2997)
  line L952 (165.41, 100.2997) -> (169.176, 100.2997)
  spline S257 degree 3 poles (169.176, 100.2997) (170.1441, 100.2997) (171.2447, 100.1395) (172.1332, 100.0667) knots 0 0 0 0 1 1 1 1
  line L953 (172.1332, 100.0667) -> (172.1332, 100.1104)
  line L954 (172.1332, 100.1104) -> (170.2767, 100.9699)
  line L955 (170.2767, 100.9699) -> (165.41, 103.49)
  line L956 (165.41, 103.49) -> (165.41, 105.2672)
  line L957 (165.41, 105.2672) -> (174.0825, 105.2672)
  line L958 (174.0825, 87.9872) -> (174.0825, 80.9658)
  line L959 (174.0825, 80.9658) -> (172.783, 80.9658)
  line L960 (172.783, 80.9658) -> (172.783, 85.9187)
  line L961 (172.783, 85.9187) -> (166.3382, 81.0241)
  line L962 (166.3382, 81.0241) -> (165.41, 81.0241)
  line L963 (165.41, 81.0241) -> (165.41, 87.5502)
  line L964 (165.41, 87.5502) -> (166.6963, 87.5502)
  line L965 (166.6963, 87.5502) -> (166.6963, 83.1072)
  line L966 (166.6963, 83.1072) -> (173.1543, 87.9872)
  line L967 (173.1543, 87.9872) -> (174.0825, 87.9872)
  line L968 (174.0825, 69.9498) -> (174.0825, 68.0706)
  line L969 (174.0825, 68.0706) -> (171.006, 67.3422)
  spline S258 degree 3 poles (171.006, 67.3422) (170.4623, 67.2111) (169.9187, 67.1383) (169.3882, 67.0509) knots 0 0 0 0 1 1 1 1
  line L970 (169.3882, 67.0509) -> (169.3882, 67.0072)
  spline S259 degree 3 poles (169.3882, 67.0072) (169.9187, 66.9489) (170.4623, 66.8324) (171.006, 66.7012) knots 0 0 0 0 1 1 1 1
  line L971 (171.006, 66.7012) -> (174.0825, 65.9583)
  line L972 (174.0825, 65.9583) -> (174.0825, 64.05)
  line L973 (174.0825, 64.05) -> (165.41, 62.7681)
  line L974 (165.41, 62.7681) -> (165.41, 64.4724)
  line L975 (165.41, 64.4724) -> (170.4358, 64.9386)
  spline S260 degree 3 poles (170.4358, 64.9386) (171.1519, 64.9969) (171.6956, 65.0114) (172.5178, 65.0551) knots 0 0 0 0 1 1 1 1
  line L976 (172.5178, 65.0551) -> (172.5178, 65.1134)
  spline S261 degree 3 poles (172.5178, 65.1134) (171.6956, 65.2591) (171.1519, 65.3902) (170.4358, 65.5795) knots 0 0 0 0 1 1 1 1
  line L977 (170.4358, 65.5795) -> (167.6245, 66.3225)
  line L978 (167.6245, 66.3225) -> (167.6245, 67.5898)
  line L979 (167.6245, 67.5898) -> (170.4358, 68.3765)
  spline S262 degree 3 poles (170.4358, 68.3765) (171.1652, 68.5513) (171.7088, 68.6824) (172.5178, 68.8426) knots 0 0 0 0 1 1 1 1
  line L980 (172.5178, 68.8426) -> (172.5178, 68.8863)
  spline S263 degree 3 poles (172.5178, 68.8863) (171.7088, 68.9155) (171.1652, 68.9591) (170.4358, 69.0174) knots 0 0 0 0 1 1 1 1
  line L981 (170.4358, 69.0174) -> (165.41, 69.4982)
  line L982 (165.41, 69.4982) -> (165.41, 71.3045)
  line L983 (165.41, 71.3045) -> (174.0825, 69.9498)
  spline S264 degree 3 poles (174.2417, 49.567) (174.2417, 47.3528) (172.6106, 45.8232) (169.7065, 45.8232) knots 0 0 0 0 1 1 1 1
  spline S265 degree 3 poles (169.7065, 45.8232) (166.8554, 45.8232) (165.2508, 47.3527) (165.2508, 49.567) knots 0 0 0 0 1 1 1 1
  spline S266 degree 3 poles (165.2508, 49.567) (165.2508, 51.7812) (166.8554, 53.3108) (169.7065, 53.3108) knots 0 0 0 0 1 1 1 1
  spline S267 degree 3 poles (169.7065, 53.3108) (172.6106, 53.3108) (174.2417, 51.7812) (174.2417, 49.567) knots 0 0 0 0 1 1 1 1
  spline S268 degree 3 poles (172.9023, 49.567) (172.9023, 50.7906) (171.7486, 51.5772) (169.7065, 51.5772) knots 0 0 0 0 1 1 1 1
  spline S269 degree 3 poles (169.7065, 51.5772) (167.7174, 51.5772) (166.5902, 50.7906) (166.5902, 49.567) knots 0 0 0 0 1 1 1 1
  spline S270 degree 3 poles (166.5902, 49.567) (166.5902, 48.3433) (167.7174, 47.5567) (169.7065, 47.5567) knots 0 0 0 0 1 1 1 1
  spline S271 degree 3 poles (169.7065, 47.5567) (171.7486, 47.5567) (172.9023, 48.3433) (172.9023, 49.567) knots 0 0 0 0 1 1 1 1
  spline S272 degree 3 poles (164.6939, 51.0383) (164.6939, 50.5139) (164.3491, 50.1351) (163.8717, 50.1351) knots 0 0 0 0 1 1 1 1
  spline S273 degree 3 poles (163.8717, 50.1351) (163.3943, 50.1351) (163.0495, 50.5139) (163.0495, 51.0383) knots 0 0 0 0 1 1 1 1
  spline S274 degree 3 poles (163.0495, 51.0383) (163.0495, 51.5627) (163.3943, 51.9414) (163.8717, 51.9414) knots 0 0 0 0 1 1 1 1
  spline S275 degree 3 poles (163.8717, 51.9414) (164.3491, 51.9414) (164.6939, 51.5627) (164.6939, 51.0383) knots 0 0 0 0 1 1 1 1
  spline S276 degree 3 poles (164.6939, 48.0957) (164.6939, 47.5712) (164.3491, 47.1925) (163.8717, 47.1925) knots 0 0 0 0 1 1 1 1
  spline S277 degree 3 poles (163.8717, 47.1925) (163.3943, 47.1925) (163.0495, 47.5712) (163.0495, 48.0957) knots 0 0 0 0 1 1 1 1
  spline S278 degree 3 poles (163.0495, 48.0957) (163.0495, 48.6201) (163.3943, 48.9989) (163.8717, 48.9989) knots 0 0 0 0 1 1 1 1
  spline S279 degree 3 poles (163.8717, 48.9989) (164.3491, 48.9989) (164.6939, 48.6201) (164.6939, 48.0957) knots 0 0 0 0 1 1 1 1
  line L984 (174.0825, 34.7197) -> (174.0825, 28.5723)
  line L985 (174.0825, 28.5723) -> (172.783, 28.5723)
  line L986 (172.783, 28.5723) -> (172.783, 33.0445)
  line L987 (172.783, 33.0445) -> (165.41, 33.0445)
  line L988 (165.41, 33.0445) -> (165.41, 34.7197)
  line L989 (165.41, 34.7197) -> (174.0825, 34.7197)
  line L990 (174.0825, 17.2649) -> (174.0825, 15.5751)
  line L991 (174.0825, 15.5751) -> (170.4623, 15.5751)
  line L992 (170.4623, 15.5751) -> (170.4623, 11.8313)
  line L993 (170.4623, 11.8313) -> (169.1628, 11.8313)
  line L994 (169.1628, 11.8313) -> (169.1628, 15.5751)
  line L995 (169.1628, 15.5751) -> (166.7095, 15.5751)
  line L996 (166.7095, 15.5751) -> (166.7095, 11.1758)
  line L997 (166.7095, 11.1758) -> (165.41, 11.1758)
  line L998 (165.41, 11.1758) -> (165.41, 17.2649)
  line L999 (165.41, 17.2649) -> (174.0825, 17.2649)
  line L1000 (193.125, 192.8033) -> (193.125, 185.7819)
  line L1001 (193.125, 185.7819) -> (191.8255, 185.7819)
  line L1002 (191.8255, 185.7819) -> (191.8255, 190.7347)
  line L1003 (191.8255, 190.7347) -> (185.3807, 185.8401)
  line L1004 (185.3807, 185.8401) -> (184.4525, 185.8401)
  line L1005 (184.4525, 185.8401) -> (184.4525, 192.3663)
  line L1006 (184.4525, 192.3663) -> (185.7388, 192.3663)
  line L1007 (185.7388, 192.3663) -> (185.7388, 187.9232)
  line L1008 (185.7388, 187.9232) -> (192.1968, 192.8033)
  line L1009 (192.1968, 192.8033) -> (193.125, 192.8033)
  line L1010 (193.125, 174.7221) -> (193.125, 168.4728)
  line L1011 (193.125, 168.4728) -> (191.8255, 168.4728)
  line L1012 (191.8255, 168.4728) -> (191.8255, 173.0323)
  line L1013 (191.8255, 173.0323) -> (189.2661, 173.0323)
  line L1014 (189.2661, 173.0323) -> (189.2661, 169.2885)
  line L1015 (189.2661, 169.2885) -> (187.9666, 169.2885)
  line L1016 (187.9666, 169.2885) -> (187.9666, 173.0323)
  line L1017 (187.9666, 173.0323) -> (185.752, 173.0323)
  line L1018 (185.752, 173.0323) -> (185.752, 168.6184)
  line L1019 (185.752, 168.6184) -> (184.4524, 168.6184)
  line L1020 (184.4524, 168.6184) -> (184.4524, 174.7221)
  line L1021 (184.4524, 174.7221) -> (193.125, 174.7221)
  line L1022 (193.125, 157.7044) -> (193.125, 156.0146)
  line L1023 (193.125, 156.0146) -> (189.2794, 156.0146)
  line L1024 (189.2794, 156.0146) -> (189.2794, 152.7515)
  line L1025 (189.2794, 152.7515) -> (193.125, 152.7515)
  line L1026 (193.125, 152.7515) -> (193.125, 151.0617)
  line L1027 (193.125, 151.0617) -> (184.4525, 151.0617)
  line L1028 (184.4525, 151.0617) -> (184.4525, 152.7515)
  line L1029 (184.4525, 152.7515) -> (187.9401, 152.7515)
  line L1030 (187.9401, 152.7515) -> (187.9401, 156.0146)
  line L1031 (187.9401, 156.0146) -> (184.4525, 156.0146)
  line L1032 (184.4525, 156.0146) -> (184.4525, 157.7044)
  line L1033 (184.4525, 157.7044) -> (193.125, 157.7044)
  line L1034 (193.125, 140.2059) -> (193.125, 138.5889)
  line L1035 (193.125, 138.5889) -> (189.3324, 138.5889)
  spline S280 degree 3 poles (189.3324, 138.5889) (188.3644, 138.5889) (187.3301, 138.7492) (186.4018, 138.822) knots 0 0 0 0 1 1 1 1
  line L1036 (186.4018, 138.822) -> (186.4018, 138.7783)
  line L1037 (186.4018, 138.7783) -> (188.2451, 137.9188)
  line L1038 (188.2451, 137.9188) -> (193.125, 135.3987)
  line L1039 (193.125, 135.3987) -> (193.125, 133.6215)
  line L1040 (193.125, 133.6215) -> (184.4525, 133.6215)
  line L1041 (184.4525, 133.6215) -> (184.4525, 135.2384)
  line L1042 (184.4525, 135.2384) -> (188.2185, 135.2384)
  spline S281 degree 3 poles (188.2185, 135.2384) (189.1866, 135.2384) (190.2872, 135.0782) (191.1757, 135.0054) knots 0 0 0 0 1 1 1 1
  line L1043 (191.1757, 135.0054) -> (191.1757, 135.0491)
  line L1044 (191.1757, 135.0491) -> (189.3192, 135.9085)
  line L1045 (189.3192, 135.9085) -> (184.4525, 138.4287)
  line L1046 (184.4525, 138.4287) -> (184.4525, 140.2059)
  line L1047 (184.4525, 140.2059) -> (193.125, 140.2059)